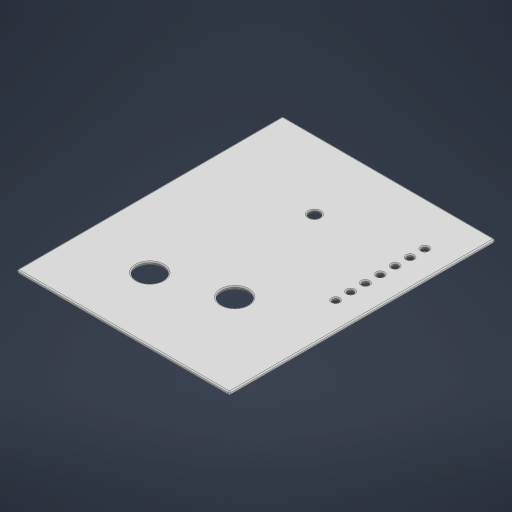
# Autodesk Inventor part: pages_extra
Saved by Autodesk Inventor 2023 (Build 270158000, 158)
## iProperties
Created: 2022-12-04
Part Number: pages_extra
Material: Generic
Document SubType Name: Modeling
Designer: jeff7
Density: 1 g/cm^3
Appearance: Default
Author: jeff7
Autodesk Inventor part; units mm, degrees
ref_plane "YZ Plane" through (0, 0, 0) normal (1, 0, 0) x (0, 1, 0)
ref_plane "XZ Plane" through (0, 0, 0) normal (0, 1, 0) x (-1, 0, 0)
ref_plane "XY Plane" through (0, 0, 0) normal (0, 0, 1) x (1, 0, 0)
sketch "page_lines" plane through (0, 0, 0) normal (0, 1, 0) x (-1, 0, 0)
  line L0 (0, 0) -> (-200, 0)
  line L1 (-200, 0) -> (-200, -250)
  line L2 (-200, -250) -> (0, -250)
  line L3 (0, -250) -> (0, 0)
  circle A0 centre (-65, -60) radius 6
  circle A1 centre (-125, -80) radius 6
  circle A2 centre (-65, -60) radius 12.5
  circle A3 centre (-65, -60) radius 8.5
  circle A4 centre (-125, -80) radius 8.5
  circle A5 centre (-125, -80) radius 12.5
  circle A6 centre (-175, -125) radius 3
  line L4 (-175, -125) -> (-175, -209)
  line L5 (-175, -125) -> (-91, -125) construction
  circle A7 centre (-175, -139) radius 3
  circle A8 centre (-175, -153) radius 3
  circle A9 centre (-175, -167) radius 3
  circle A10 centre (-175, -181) radius 3
  circle A11 centre (-175, -195) radius 3
  circle A12 centre (-175, -209) radius 3
  circle A13 centre (-95, -185) radius 2.5
  circle A14 centre (-95, -185) radius 5
  point P0 (-200, -125)
  dimension "d0" = 200
  dimension "d1" = 250
  dimension "d2" = 12
  dimension "d3" = 12
  dimension "d4" = 25
  dimension "d5" = 17
  dimension "d6" = 17
  dimension "d7" = 25
  dimension "d8" = 75
  dimension "d9" = 80
  dimension "d10" = 65
  dimension "d11" = 60
  dimension "d12" = 6
  dimension "d13" = 84
  dimension "d14" = 90
  dimension "d15" = 25
  dimension "d16" = 125
  dimension "d19" = 14
  dimension "d24" = 5
  dimension "d25" = 10
  dimension "d26" = 65
  dimension "d27" = 95
  constraints: 15 centre point, 12 end point, 5 coincident, 2 horizontal, 2 parallel, 2 perpendicular, 2 vertical, 1 midpoint, 12 other
  measures "d0" distance of L2.end L1.end
  measures "d1" distance of L1.end L0.end
  measures "d2" diameter of A0
  measures "d3" diameter of A1
  measures "d4" diameter of A2
  measures "d5" diameter of A3
  measures "d6" diameter of A4
  measures "d7" diameter of A5
  measures "d8" distance from line of L1 A1.centre
  measures "d9" distance from line of L0 A1.centre
  measures "d10" distance from line of L3 A0.centre
  measures "d11" distance from line of L0 A0.centre
  measures "d12" diameter of A6
  measures "d13" distance of L4.start L4.end
  measures "d14" angle of L4 L5
  measures "d15" distance of point (-200, -125) L4.start
  measures "d16" distance from line of L0 L4.start
  measures "d19" distance of L4.start A7.centre
  measures "d24" diameter of A13
  measures "d25" diameter of A14
  measures "d26" distance from line of L2 A13.centre
  measures "d27" distance from line of L3 A13.centre
extrude "extra" add sketch "page_lines" along normal blind 3 contours L3 L2 L1 L0
fillet "Fillet1" radius 1 32 edges at (77.5, 3, -60) (77.5, 0, -60) (100, 3, -185) (100, 0, -185) (178, 3, -125) (178, 0, -125) (200, 3, -125) (200, 0, -125) (100, 0, 0) (100, 3, 0) (200, 1.5, 0) (0, 1.5, 0) (0, 3, -125) (0, 0, -125) (0, 1.5, -250) (100, 3, -250) (100, 0, -250) (200, 1.5, -250) (178, 3, -139) (178, 0, -139) (137.5, 3, -80) (137.5, 0, -80) (178, 3, -153) (178, 0, -153) (178, 3, -167) (178, 0, -167) (178, 3, -181) (178, 0, -181) (178, 0, -195) (178, 3, -195) (178, 0, -209) (178, 3, -209)
body "Solid1"
